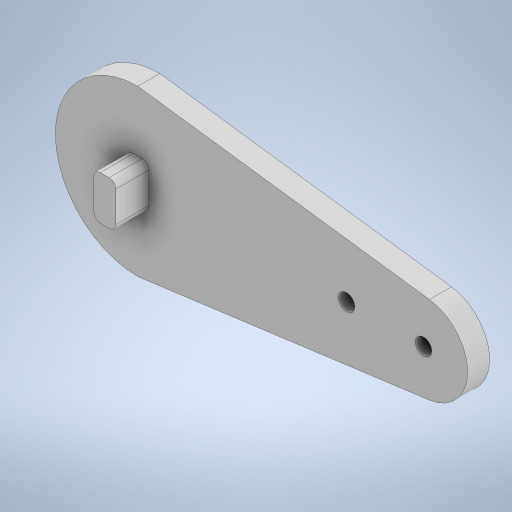
# Autodesk Inventor part: tweaker
Saved by Autodesk Inventor 2024.2 (Build 282272000, 272)
## iProperties
Created: 2024-01-09
Part Number: tweaker
Material: PLA
Document SubType Name: Modeling
Designer: Konrad
Density: 1 g/cm^3
Appearance: Domyślna
Author: Konrad
Autodesk Inventor part; units mm, degrees
ref_plane "YZ Plane" through (0, 0, 0) normal (1, 0, 0) x (0, 1, 0)
ref_plane "XZ Plane" through (0, 0, 0) normal (0, 1, 0) x (-1, 0, 0)
ref_plane "XY Plane" through (0, 0, 0) normal (0, 0, 1) x (1, 0, 0)
sketch "Szkic1" plane through (0, 0, 0) normal (0, 0, 1) x (1, 0, 0)
  circle A0 centre (0, 0) radius 7.5 construction
  line L0 (0, 7.5) -> (30, 7.5)
  line L1 (30, 7.5) -> (30, -7.5)
  line L2 (30, -7.5) -> (0, -7.5)
  line L3 (0, -7.5) -> (0, 7.5) construction
  arc A1 (0, 7.5) -> (0, -7.5) centre (0, 0) ccw
  line L4 (-1, -2) -> (1, -2)
  line L5 (1, -2) -> (1, 2)
  line L6 (1, 2) -> (-1, 2)
  line L7 (-1, 2) -> (-1, -2)
  line L8 (-1, -2) -> (1, 2) construction
  line L9 (1, -2) -> (-1, 2) construction
  circle A2 centre (26, 0) radius 4
  line L10 (-15, 0) -> (37.5, 0) construction
  line L11 (0, 7.5) -> (26.5284, 3.965)
  line L12 (0, -7.5) -> (26.5284, -3.965)
  circle A3 centre (26, 0) radius 0.75
  circle A4 centre (19, 0) radius 0.75
  point P0 (30, 0)
  dimension "d0" = 15
  dimension "d1" = 2
  dimension "d2" = 4
  dimension "d3" = 30
  dimension "d8" = 8
  dimension "d9" = 1.5
  dimension "d10" = 1.5
  dimension "d11" = 7
  dimension "d12" = 19
  constraints: 24 end point, 7 point on circle, 5 centre point, 5 midpoint, 4 parallel, 3 coincident, 2 horizontal, 2 perpendicular, 2 point on line, 2 tangent
  measures "d0" diameter of A0
  measures "d1" distance of L6.end L5.end
  measures "d2" distance of L5.end L4.end
  measures "d3" distance of L0.start L0.end
  measures "d8" diameter of A2
  measures "d9" diameter of A3
  measures "d10" diameter of A4
  measures "d11" distance of A2.centre A4.centre
  measures "d12" distance of A4.centre point (0, 0)
extrude "Wyciągnięcie proste1" add sketch "Szkic1" against normal blind 2 contours L11 A2 L12 A1 | A2 | L7 L6 L5 L4
extrude "Wyciągnięcie proste2" add sketch "Szkic1" along normal blind 3 contours L7 L6 L5 L4
fillet "Zaokrąglenie1" radius 0.6 4 edges at (-1, -2, 1.5) (1, -2, 1.5) (-1, 2, 1.5) (1, 2, 1.5)
